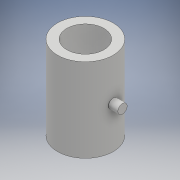
# Autodesk Inventor part: стакан_v1
Saved by Autodesk Inventor 2017.3 (Build 213256000, 256)
## iProperties
Part Number: стакан_v1
Material: Типовые
Document SubType Name: Modeling
Designer: Alexnav
Density: 1 g/cm^3
Appearance: По умолчанию
Mass: 126.457 g
Surface Area: 285.946 cm^2
Volume: 126.457 cm^3
Author: Alexnav
Autodesk Inventor part; units mm, degrees
ref_plane "YZ Plane" through (0, 0, 0) normal (1, 0, 0) x (0, 1, 0)
ref_plane "XZ Plane" through (0, 0, 0) normal (0, 1, 0) x (-1, 0, 0)
ref_plane "XY Plane" through (0, 0, 0) normal (0, 0, 1) x (1, 0, 0)
sketch "Эскиз1" plane through (0, 0, 0) normal (0, 0, 1) x (1, 0, 0)
  circle A0 centre (0, 0) radius 20
  circle A1 centre (0, 0) radius 30
  dimension "d0" = 40
  dimension "d1" = 10
  constraints: 2 centre point, 2 coincident
  measures "d0" diameter of A0
  measures "d1" radial gap between concentric circles of A1 A0
extrude "Выдавливание1" add sketch "Эскиз1" along normal mid plane 90
ref_plane "РабПлоскость1" through (30, 0, 0) normal (1, 0, 0) x (0, 1, 0)
sketch "Эскиз4" plane through (30, 0, 0) normal (1, 0, 0) x (0, 1, 0)
  circle A0 centre (0, 0) radius 5
  dimension "d5" = 10
  constraints: 1 centre point, 1 coincident
  measures "d5" diameter of A0
extrude "Выдавливание2" add sketch "Эскиз4" against normal up to surface round surface about axis through (0, 0, 0) along (0, 0, 1) radius 30 far side no
sketch "Эскиз6" plane through (30, 0, 0) normal (1, 0, 0) x (0, 0, -1)
  arc A0 (5, 0) -> (-5, 0) centre (0, 0) ccw projected
  circle A1 centre (0, 0) radius 4.9989
  point P0 (-10, 0)
  point P1 (10, 0)
  constraints: 2 horizontal alignment, 1 centre point, 1 coincident, 1 other
extrude "Выдавливание3" add sketch "Эскиз6" along normal blind 10
